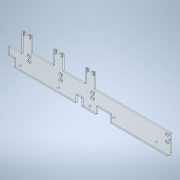
# Autodesk Inventor part: 104.002.01_Foerderband_Halterung_hinten
Saved by Autodesk Inventor 2021 (Build 250183000, 183)
## iProperties
Created: 2020-11-24
Part Number: 104.002.01_Foerderband_Halterung_hinten
Material: Generic
Document SubType Name: Modeling
Designer: Alexander Fritzsche
Density: 1 g/cm^3
Appearance: Default
Author: Alexander Fritzsche
Autodesk Inventor part; units mm, degrees
ref_plane "YZ Plane" through (0, 0, 0) normal (1, 0, 0) x (0, 1, 0)
ref_plane "XZ Plane" through (0, 0, 0) normal (0, 1, 0) x (-1, 0, 0)
ref_plane "XY Plane" through (0, 0, 0) normal (0, 0, 1) x (1, 0, 0)
sketch "Sketch1" plane through (0, 0, 0) normal (0, 0, 1) x (1, 0, 0)
  line L0 (308.15, 40) -> (308.15, -25)
  line L1 (-308.15, -25) -> (-308.15, 18)
  line L2 (0, 136.1557) -> (0, 0)
  line L3 (0, 0) -> (214.7287, 0)
  line L4 (-218.75, 40) -> (-218.75, 95)
  line L5 (-218.75, 95) -> (-253.75, 95)
  line L6 (-253.75, 95) -> (-253.75, 18)
  line L7 (-98.75, 40) -> (-98.75, 95)
  line L8 (-98.75, 95) -> (-133.75, 95)
  line L9 (-133.75, 95) -> (-133.75, 40)
  line L10 (21.25, 40) -> (21.25, 95)
  line L11 (21.25, 95) -> (-13.75, 95)
  line L12 (-13.75, 95) -> (-13.75, 40)
  line L13 (-218.75, 40) -> (-133.75, 40)
  line L14 (-98.75, 40) -> (-13.75, 40)
  line L15 (21.25, 40) -> (308.15, 40)
  arc A0 (-308.15, -25) -> (-293.15, -40) centre (-293.15, -25) ccw
  arc A1 (293.15, -40) -> (308.15, -25) centre (293.15, -25) ccw
  line L16 (293.15, -40) -> (252.5, -40)
  line L17 (-257.5, -40) -> (-293.15, -40)
  line L18 (287.95, 30.2) -> (298.35, 30.2)
  line L19 (298.35, 30.2) -> (298.35, 24.8)
  line L20 (298.35, 24.8) -> (287.95, 24.8)
  line L21 (287.95, 24.8) -> (287.95, 30.2)
  line L22 (287.95, 5.2) -> (298.35, 5.2)
  line L23 (298.35, 5.2) -> (298.35, -0.2)
  line L24 (298.35, -0.2) -> (287.95, -0.2)
  line L25 (287.95, -0.2) -> (287.95, 5.2)
  line L26 (252.5, -40) -> (-257.5, -40)
  line L27 (88.15, -10) -> (88.15, -40)
  line L28 (21.15, -40) -> (21.15, -10)
  line L29 (-18.85, -10) -> (-18.85, -40)
  line L30 (-283.15, -40) -> (-283.15, -10)
  line L31 (-283.15, -10) -> (-308.15, -10)
  line L32 (88.15, -10) -> (21.15, -10)
  line L33 (-18.85, -10) -> (-98.85, -10)
  line L34 (-98.85, -10) -> (-98.85, -40)
  circle A2 centre (-263.15, -25) radius 2.65
  circle A3 centre (-118.85, -25) radius 2.65
  circle A4 centre (1.15, -25) radius 2.65
  line L35 (-247.75, 91) -> (-247.75, 83) construction
  line L36 (-249.5, 91) -> (-249.5, 83)
  line L37 (-246, 83) -> (-246, 91)
  arc A5 (-246, 91) -> (-249.5, 91) centre (-247.75, 91) ccw
  arc A6 (-249.5, 83) -> (-246, 83) centre (-247.75, 83) ccw
  line L38 (-224.75, 91) -> (-224.75, 83) construction
  line L39 (-226.5, 91) -> (-226.5, 83)
  line L40 (-223, 83) -> (-223, 91)
  arc A7 (-223, 91) -> (-226.5, 91) centre (-224.75, 91) ccw
  arc A8 (-226.5, 83) -> (-223, 83) centre (-224.75, 83) ccw
  line L41 (-236.25, 95) -> (-236.25, 40) construction
  line L42 (-126, 83) -> (-126, 91)
  line L43 (-127.75, 91) -> (-127.75, 83) construction
  arc A9 (-129.5, 83) -> (-126, 83) centre (-127.75, 83) ccw
  line L44 (-129.5, 91) -> (-129.5, 83)
  arc A10 (-126, 91) -> (-129.5, 91) centre (-127.75, 91) ccw
  line L45 (-103, 83) -> (-103, 91)
  arc A11 (-106.5, 83) -> (-103, 83) centre (-104.75, 83) ccw
  line L46 (-104.75, 91) -> (-104.75, 83) construction
  line L47 (-106.5, 91) -> (-106.5, 83)
  arc A12 (-103, 91) -> (-106.5, 91) centre (-104.75, 91) ccw
  line L48 (-6, 83) -> (-6, 91)
  line L49 (-7.75, 91) -> (-7.75, 83) construction
  arc A13 (-9.5, 83) -> (-6, 83) centre (-7.75, 83) ccw
  line L50 (-9.5, 91) -> (-9.5, 83)
  arc A14 (-6, 91) -> (-9.5, 91) centre (-7.75, 91) ccw
  line L51 (17, 83) -> (17, 91)
  arc A15 (13.5, 83) -> (17, 83) centre (15.25, 83) ccw
  line L52 (15.25, 91) -> (15.25, 83) construction
  line L53 (13.5, 91) -> (13.5, 83)
  arc A16 (17, 91) -> (13.5, 91) centre (15.25, 91) ccw
  circle A17 centre (-236.25, 98) radius 9.25
  line L54 (-98.75, 40) -> (-98.75, 95)
  circle A18 centre (-116.25, 98) radius 9.25
  line L55 (21.25, 40) -> (21.25, 95)
  circle A19 centre (3.75, 98) radius 9.25
  line L56 (-253.75, 18) -> (-308.15, 18)
  point P0 (-247.75, 87)
  point P1 (-224.75, 87)
  point P2 (-127.75, 87)
  point P3 (-104.75, 87)
  point P4 (-7.75, 87)
  point P5 (15.25, 87)
  point P6 (-107.5, 95)
  point P7 (-125, 95)
  point P8 (-227.5, 95)
  point P9 (-245, 95)
  point P10 (12.5, 95)
  point P11 (-5, 95)
  dimension "d2" = 54.4
  dimension "d3" = 35
  dimension "d4" = 85
  dimension "d5" = 55
  dimension "d6" = 15
  dimension "d10" = 80
  dimension "d99" = 5.4
  dimension "d101" = 10.4
  dimension "d102" = 9.8
  dimension "d103" = 19.6
  dimension "d104" = 9.8
  dimension "d175" = 220
  dimension "d176" = 67
  dimension "d177" = 40
  dimension "d178" = 25
  dimension "d181" = 80
  dimension "d182" = 30
  dimension "d183" = 15
  dimension "d184" = 20
  dimension "d185" = 20
  dimension "d186" = 5.3
  dimension "d187" = 5.3
  dimension "d188" = 5.3
  dimension "d189" = 20
  dimension "d193" = 3.5
  dimension "d194" = 3.5
  dimension "d195" = 8
  dimension "d196" = 8
  dimension "d197" = 4
  dimension "d198" = 4
  dimension "d202" = 120
  dimension "d207" = 18.5
  dimension "d208" = 3
  dimension "d209" = 17.5
  dimension "d212" = 120
  dimension "d230" = 616.3
  dimension "d231" = 22
  dimension "d285" = 11.5
  constraints: 126 end point, 28 point on circle, 20 centre point, 17 parallel, 14 tangent, 12 horizontal, 12 perpendicular, 10 point on line, 8 collinear, 6 vertical, 3 midpoint, 2 horizontal alignment, 1 equal radius, 61 other
  measures "d2" distance between parallel lines of L6 L1
  measures "d3" distance of L4.end L5.end
  measures "d4" distance of L4.start L9.end
  measures "d5" distance between parallel lines of L13 L5
  measures "d6" radius of A0
  measures "d10" distance between parallel lines of L15 L16
  measures "d99" distance of L18.end L19.end
  measures "d101" distance of L18.start L18.end
  measures "d102" distance between parallel lines of L15 L18
  measures "d103" distance between parallel lines of L22 L20
  measures "d104" distance between parallel lines of L0 L23
  measures "d175" distance between parallel lines of L0 L27
  measures "d176" distance between parallel lines of L27 L28
  measures "d177" distance between parallel lines of L28 L29
  measures "d178" distance between parallel lines of L1 L30
  measures "d181" distance between parallel lines of L29 L34
  measures "d182" distance between parallel lines of L26 L32
  measures "d183" distance from line of L26 A2.centre
  measures "d184" distance from line of L30 A2.centre
  measures "d185" distance from line of L34 A3.centre
  measures "d186" diameter of A3
  measures "d187" diameter of A2
  measures "d188" diameter of A4
  measures "d189" distance from line of L29 A4.centre
  measures "d193" distance between parallel lines of L37 L36
  measures "d194" distance between parallel lines of L40 L39
  measures "d195" distance of L35.start L35.end
  measures "d196" distance of L38.start L38.end
  measures "d197" distance from line of L5 L38.start
  measures "d198" distance from line of L5 L35.start
  measures "d202" distance of L37.end L42.end
  measures "d207" diameter of A17
  measures "d208" distance from line of L5 A17.centre
  measures "d209" distance from line of L4 A17.centre
  measures "d212" distance of L4.start L54.start
  measures "d230" distance between parallel lines of L0 L1
  measures "d231" distance between parallel lines of L56 L13
  measures "d285" distance between parallel lines of L41 L38
extrude "Extrusion1" add sketch "Sketch1" along normal blind 5 contours L0 A1 L16 L26 L27 L32 L28 L29 L33 L34 L17 L30 L31 L1 L56 L6 L5 A17 L4 L13 L9 L8 A18 L7 L14 L12 L11 A19 L10 L15 | L26 L28 L32 L27 | L26 L34 L33 L29
fillet "Fillet1" radius 2 16 edges at (-253.75, 95, 2.5) (-253.75, 18, 2.5) (-308.15, 18, 2.5) (308.15, 40, 2.5) (21.25, 95, 2.5) (21.25, 40, 2.5) (-13.75, 95, 2.5) (-13.75, 40, 2.5) (-98.75, 40, 2.5) (-98.75, 95, 2.5) (-133.75, 95, 2.5) (-133.75, 40, 2.5) (-218.75, 40, 2.5) (-218.75, 95, 2.5) (-308.15, -10, 2.5) (-283.15, -10, 2.5)
sketch "Sketch11" plane through (0, 0, 5) normal (0, 0, 1) x (1, 0, 0)
  line L0 (308.15, -25) -> (308.15, 38) projected
  line L1 (298.35, 24.8) -> (287.95, 24.8) projected
  point P0 (0, 0)
  point P1 (302.15, 15)
  point P2 (308.15, 38)
  point P3 (312.5, -10)
  dimension "d140" = 6
  dimension "d141" = 9.8
  constraints: 1 other
  measures "d141" distance from line of L1 point (302.15, 15)
hole "Hole10" at (302.15, 15, 5) direction (0, 0, -1) diameter 5.5 end through all
sketch "Skizze13" plane through (0, 0, 5) normal (0, 0, 1) x (1, 0, 0)
  line L0 (-283.15, -40) -> (293.15, -40) projected
  line L1 (-49.15, -12) -> (-27.15, -12)
  line L2 (-27.15, -12) -> (-27.15, -40)
  line L3 (-27.15, -40) -> (-49.15, -40)
  line L4 (-49.15, -40) -> (-49.15, -12)
  line L5 (-308.15, 16) -> (-308.15, -8) projected
  line L6 (26.85, -12) -> (81.85, -12)
  line L7 (81.85, -12) -> (81.85, -40)
  line L8 (81.85, -40) -> (26.85, -40)
  line L9 (26.85, -40) -> (26.85, -12)
  point P0 (0, 0)
  point P1 (-49.15, -40)
  point P2 (26.85, -40)
  dimension "d232" = 22
  dimension "d233" = 28
  dimension "d234" = 259
  dimension "d238" = 335
  dimension "d239" = 55
  constraints: 16 end point, 4 parallel, 3 point on line, 2 horizontal, 2 perpendicular
  measures "d232" distance between parallel lines of L2 L4
  measures "d233" distance between parallel lines of L0 L1
  measures "d234" distance between parallel lines of L5 L4
  measures "d238" distance between parallel lines of L5 L9
  measures "d239" distance between parallel lines of L7 L9
extrude "Extrusion3" cut sketch "Skizze13" against normal through all
fillet "Rundung6" radius 2 4 edges at (-49.15, -12, 2.5) (-27.15, -12, 2.5) (26.85, -12, 2.5) (81.85, -12, 2.5)
sketch "Skizze14" plane through (0, 0, 5) normal (0, 0, 1) x (1, 0, 0)
  line L0 (-308.15, 16) -> (-308.15, -8) projected
  line L1 (83.85, -40) -> (293.15, -40) projected
  point P0 (0, 0)
  point P1 (251.85, -18)
  point P2 (91.85, -18)
  dimension "d241" = 560
  dimension "d242" = 22
  dimension "d243" = 160
  measures "d241" distance from line of L0 point (251.85, -18)
  measures "d242" distance from line of L1 point (251.85, -18)
  measures "d243" distance of point (91.85, -18) point (251.85, -18)
hole "Bohrung11" at (251.85, -18, 5) at (91.85, -18, 5) direction (0, 0, -1) diameter 4.5 end through all
sketch "Skizze16" plane through (0, 0, 5) normal (0, 0, 1) x (1, 0, 0)
  line L0 (-233.95, 26.75) -> (-223.75, 26.75)
  line L1 (-223.75, 26.75) -> (-223.75, 20.55)
  line L2 (-223.75, 20.55) -> (-233.95, 20.55)
  line L3 (-233.95, 20.55) -> (-233.95, 26.75)
  line L4 (-233.95, 7.55) -> (-223.75, 7.55)
  line L5 (-223.75, 7.55) -> (-223.75, 1.35)
  line L6 (-223.75, 1.35) -> (-233.95, 1.35)
  line L7 (-233.95, 1.35) -> (-233.95, 7.55)
  line L8 (-218.75, 42) -> (-218.75, 93) projected
  line L9 (-135.75, 40) -> (-216.75, 40) projected
  circle A0 centre (-228.85, 14.05) radius 1.75
  line L10 (-113.95, 26.75) -> (-103.75, 26.75)
  line L11 (-103.75, 26.75) -> (-103.75, 20.55)
  line L12 (-103.75, 20.55) -> (-113.95, 20.55)
  line L13 (-113.95, 20.55) -> (-113.95, 26.75)
  circle A1 centre (-108.85, 14.05) radius 1.75
  line L14 (-113.95, 7.55) -> (-103.75, 7.55)
  line L15 (-103.75, 7.55) -> (-103.75, 1.35)
  line L16 (-113.95, 1.35) -> (-113.95, 7.55)
  line L17 (-103.75, 1.35) -> (-113.95, 1.35)
  line L18 (6.05, 26.75) -> (16.25, 26.75)
  line L19 (16.25, 26.75) -> (16.25, 20.55)
  line L20 (16.25, 20.55) -> (6.05, 20.55)
  line L21 (6.05, 20.55) -> (6.05, 26.75)
  circle A2 centre (11.15, 14.05) radius 1.75
  line L22 (6.05, 7.55) -> (16.25, 7.55)
  line L23 (16.25, 7.55) -> (16.25, 1.35)
  line L24 (6.05, 1.35) -> (6.05, 7.55)
  line L25 (16.25, 1.35) -> (6.05, 1.35)
  point P0 (0, 0)
  dimension "d267" = 5
  dimension "d268" = 10.2
  dimension "d269" = 6.2
  dimension "d270" = 6.2
  dimension "d271" = 13
  dimension "d272" = 13.25
  dimension "d273" = 3.5
  dimension "d274" = 5.1
  dimension "d275" = 6.5
  dimension "d280" = 120
  constraints: 48 end point, 6 point on line, 4 parallel, 3 centre point, 3 horizontal, 2 perpendicular, 36 other
  measures "d267" distance between parallel lines of L1 L8
  measures "d268" distance of L0.start L0.end
  measures "d269" distance between parallel lines of L2 L0
  measures "d270" distance between parallel lines of L6 L4
  measures "d271" distance between parallel lines of L2 L4
  measures "d272" distance between parallel lines of L9 L0
  measures "d273" diameter of A0
  measures "d274" distance from line of L1 A0.centre
  measures "d275" distance from line of L2 A0.centre
  measures "d280" distance of L0.start L10.start
extrude "Extrusion4" cut sketch "Skizze16" against normal through all
fillet "Rundung7" radius 4 6 edges at (12.5, 95, 2.5) (-5, 95, 2.5) (-107.5, 95, 2.5) (-125, 95, 2.5) (-227.5, 95, 2.5) (-245, 95, 2.5)
sketch "Skizze17" plane through (0, 0, 5) normal (0, 0, 1) x (1, 0, 0)
  line L0 (-308.15, 18) -> (-305.15, 18)
  line L1 (-305.15, 18) -> (-305.15, -10)
  line L2 (-305.15, -10) -> (-308.15, -10)
  line L3 (-308.15, -10) -> (-308.15, 18)
  line L4 (-255.75, 18) -> (-306.15, 18) projected
  line L5 (-306.15, -10) -> (-285.15, -10) projected
  line L6 (-308.15, 16) -> (-308.15, -8) projected
  point P0 (0, 0)
  dimension "d287" = 3
  constraints: 8 end point, 3 collinear, 2 parallel, 1 horizontal, 1 perpendicular
  measures "d287" distance between parallel lines of L3 L1
extrude "Extrusion5" cut sketch "Skizze17" against normal through all
fillet "Rundung8" radius 2 2 edges at (-305.15, 18, 2.5) (-305.15, -10, 2.5)
body "Solid1"
